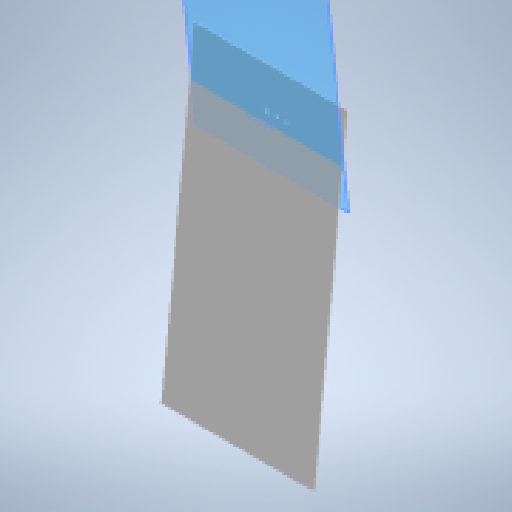
# Autodesk Inventor part: panel
Saved by Autodesk Inventor 2024.3 (Build 283343000, 343)
## iProperties
Created: 2025-05-29
Part Number: panel
Material: Generic
Document SubType Name: Modeling
Designer: Yuhsuan Chen
Density: 1 g/cm^3
Appearance: Default
Author: Yuhsuan Chen
Autodesk Inventor part; units mm, degrees
ref_plane "YZ Plane" through (0, 0, 0) normal (1, 0, 0) x (0, 1, 0)
ref_plane "XZ Plane" through (0, 0, 0) normal (0, 1, 0) x (-1, 0, 0)
ref_plane "XY Plane" through (0, 0, 0) normal (0, 0, 1) x (1, 0, 0)
sketch "Sketch2" plane through (0, 0, 0) normal (1, 0, 0) x (0, 1, 0)
  line L0 (9.7757, 0) -> (-10.7, 0) projected
  line L1 (27.1787, -1.709) -> (12.4213, -1.709) projected
  line L2 (10.7, 0) -> (9.7757, 0) projected
  arc A0 (11, -0.3) -> (10.7, 0) centre (10.7, -0.3) ccw projected
  line L3 (11, -15) -> (11, -0.3) projected
  line L4 (-229.8991, 25.4922) -> (33.0555, -2.2844)
  line L5 (72.0462, -3.8892) -> (-254.3637, 30.5904)
  line L6 (33.0555, -2.2844) -> (33.3182, 0.2018)
  line L7 (-27.0281, 6.5763) -> (-27.2907, 4.0901)
  point P0 (0, 0)
  point P1 (33.3182, 0.2018)
  dimension "d5" = 2.5
  constraints: 8 end point, 2 perpendicular, 2 point on line, 1 parallel
  measures "d5" distance between parallel lines of L4 L5
extrude "Extrusion2" add sketch "Sketch2" along normal mid plane 354.71
ref_plane "Work Plane1" through (-31.6, 28.9, -15.3) normal (0, 0, 1) x (-0.0000001, -1, 0)
sketch "Sketch3" plane through (-100, -27.0281, -15.3) normal (0, 0, 1) x (1, 0, 0)
  circle A0 centre (99.4902, 46.8281) radius 4.4577 projected
  circle A1 centre (122.9497, 46.8285) radius 3.99 projected
  line L0 (144.7507, 45.1805) -> (148.0507, 45.1805) projected
  circle A2 centre (99.4902, 46.8281) radius 6.5
  circle A3 centre (122.9497, 46.8285) radius 5
  circle A4 centre (146.4007, 46.8285) radius 3.5
  line L1 (148.0507, 48.4805) -> (144.7507, 48.4805) projected
  line L2 (144.4007, 48.8305) -> (144.4007, 44.8305) projected
  line L3 (148.0507, 45.1805) -> (148.0507, 48.4805) projected
  line L4 (144.7507, 45.1805) -> (148.0507, 45.1805) projected
  line L5 (148.0507, 48.4805) -> (144.7507, 48.4805) projected
  line L6 (144.7507, 48.4805) -> (144.7507, 45.1805) projected
  line L7 (149.6507, 50.0785) -> (143.1507, 50.0785)
  line L8 (143.1507, 50.0785) -> (143.1507, 43.5785)
  line L9 (143.1507, 43.5785) -> (149.6507, 43.5785)
  line L10 (149.6507, 43.5785) -> (149.6507, 50.0785)
  line L11 (149.6507, 50.0785) -> (143.1507, 43.5785) construction
  line L12 (143.1507, 50.0785) -> (149.6507, 43.5785) construction
  point P0 (146.4007, 45.1805)
  dimension "d13" = 13
  dimension "d14" = 10
  dimension "d15" = 7
  dimension "d20" = 6.5
  dimension "d21" = 6.5
  constraints: 12 end point, 3 centre point, 3 midpoint, 2 coincident, 2 parallel, 1 horizontal, 1 horizontal alignment, 1 perpendicular, 1 vertical alignment
  measures "d13" diameter of A2
  measures "d14" diameter of A3
  measures "d15" diameter of A4
  measures "d20" distance of L9.end L8.end
  measures "d21" distance of L8.end L7.end
extrude "Extrusion3" cut sketch "Sketch3" along normal through all contours A0 | A1 | L6 L1 L3 L0 | A2 | A3 | L10 A4 L9 L8 L7 | A4 L7 L10 | L10 L9 A4 | A4 L8 L7 | L9 L8 A4
sketch "Sketch4" plane through (-177.355, -27.2907, 4.0901) normal (0, -0.9944671, 0.1050482) x (1, 0, 0)
  line L0 (354.71, 0) -> (0, 0) projected
  line L1 (354.71, 2.5) -> (354.71, 0) projected
  line L2 (0, 2.5) -> (354.71, 2.5) projected
  line L3 (0, 0) -> (0, 2.5) projected
  point P0 (177.355, -1.2007)
extrude "Extrusion4" add sketch "Sketch4" along normal blind 600
sketch "Sketch5" plane through (-177.355, 33.3182, 0.2018) normal (0, 0.9944671, -0.1050482) x (1, 0, 0)
  line L0 (0, 0) -> (354.71, 0) projected
  line L1 (354.71, 2.5) -> (354.71, 0) projected
  line L2 (0, 2.5) -> (354.71, 2.5) projected
  line L3 (0, 0) -> (0, 2.5) projected
  point P0 (177.355, 3.7007)
extrude "Extrusion5" add sketch "Sketch5" along normal blind 72
sketch "Sketch6" plane through (-177.355, -623.7084, 69.6052) normal (0, 0.1050482, 0.9944671) x (1, 0, 0)
  point P0 (177.355, 627.5694)
body "Solid2"
